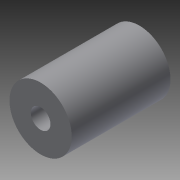
# Autodesk Inventor part: Wheel_Coupler
Saved by Autodesk Inventor 2015 (Build 190159000, 159)
## iProperties
Created: 2014-11-06
Part Number: Wheel_Coupler
Material: Generic
Document SubType Name: Modeling
Designer: bpowe_000
Density: 1 g/cm^3
Appearance: Default
Author: bpowe_000
Autodesk Inventor part; units mm, degrees
ref_plane "YZ Plane" through (0, 0, 0) normal (1, 0, 0) x (0, 1, 0)
ref_plane "XZ Plane" through (0, 0, 0) normal (0, 1, 0) x (-1, 0, 0)
ref_plane "XY Plane" through (0, 0, 0) normal (0, 0, 1) x (1, 0, 0)
sketch "Sketch1" plane through (0, 0, 0) normal (0, 1, 0) x (-1, 0, 0)
  circle A0 centre (0, 0) radius 8
  dimension "d0" = 16
  constraints: 1 centre point, 1 coincident
  measures "d0" diameter of A0
extrude "Extrusion1" add sketch "Sketch1" along normal blind 25.4
sketch "Sketch3" plane through (0, 25.4, 0) normal (0, 1, 0) x (1, 0, 0)
  line L0 (-1.61, -1.61) -> (1.61, -1.61)
  line L1 (1.61, -1.61) -> (1.61, 1.61)
  line L2 (1.61, 1.61) -> (-1.61, 1.61)
  line L3 (-1.61, 1.61) -> (-1.61, -1.61)
  point P0 (0, 0)
  dimension "d13" = 3.22
  dimension "d15" = 1.61
  dimension "d16" = 1.61
  constraints: 8 end point, 2 parallel, 2 perpendicular, 1 horizontal
  measures "d13" distance of L2.end L0.start
  measures "d15" distance from line of L0 point (0, 0)
  measures "d16" distance from line of L1 point (0, 0)
extrude "Extrusion2" cut sketch "Sketch3" against normal blind 12.7
sketch "Sketch4" plane through (0, 0, 0) normal (0, -1, 0) x (1, 0, 0)
  circle A0 centre (0, 0) radius 2.525
  dimension "d19" = 5.05
  constraints: 1 centre point, 1 coincident
  measures "d19" diameter of A0
extrude "Extrusion3" cut sketch "Sketch4" against normal blind 12.7
equation "\"d15\" = 0.5 * d13"
equation "\"d16\" = 0.5 * d13"
body "Solid1"
